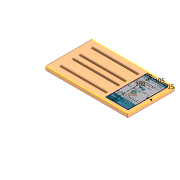
# Autodesk Inventor part: dubpen-platform
Saved by Autodesk Inventor 2020 (Build 240168000, 168)
## iProperties
Created: 2021-06-21
Part Number: dubpen-platform
Material: Generic
Document SubType Name: Modeling
Designer: Aidan Lee
Density: 1 g/cm^3
Appearance: Cherry - Natural Low Gloss
Author: Aidan Lee
Autodesk Inventor part; units mm, degrees
ref_plane "YZ Plane" through (0, 0, 0) normal (1, 0, 0) x (0, 1, 0)
ref_plane "XZ Plane" through (0, 0, 0) normal (0, 1, 0) x (-1, 0, 0)
ref_plane "XY Plane" through (0, 0, 0) normal (0, 0, 1) x (1, 0, 0)
sketch "Sketch1" plane through (0, 0, 0) normal (0, 1, 0) x (-1, 0, 0)
  line L0 (0, 0) -> (-390, 0)
  line L1 (-390, 0) -> (-390, -219)
  line L2 (-390, -219) -> (0, -219)
  line L3 (0, -219) -> (0, 0)
  line L4 (-35, -38.7) -> (-255, -38.7)
  line L5 (-255, -38.7) -> (-255, -30.7)
  line L6 (-255, -30.7) -> (-35, -30.7)
  line L7 (-35, -30.7) -> (-35, -38.7)
  line L8 (-35, -97) -> (-255, -97)
  line L9 (-255, -97) -> (-255, -89)
  line L10 (-255, -89) -> (-35, -89)
  line L11 (-35, -89) -> (-35, -97)
  line L12 (68.8158, -109.5) -> (84.9045, -109.5) construction
  line L13 (-35, -180.3) -> (-255, -180.3)
  line L14 (-255, -180.3) -> (-255, -188.3)
  line L15 (-255, -188.3) -> (-35, -188.3)
  line L16 (-35, -188.3) -> (-35, -180.3)
  line L17 (-35, -122) -> (-255, -122)
  line L18 (-255, -122) -> (-255, -130)
  line L19 (-255, -130) -> (-35, -130)
  line L20 (-35, -130) -> (-35, -122)
  point P0 (0, -109.5)
  point P1 (76.8601, -109.5)
  dimension "d0" = 219
  dimension "d1" = 50.3
  dimension "d2" = 8
  dimension "d3" = 8
  dimension "d4" = 35
  dimension "d6" = 220
  dimension "d7" = 25
  dimension "d8" = 30.7
  dimension "d9" = 30.7
  dimension "d12" = 390
  constraints: 42 end point, 8 symmetric about line, 6 parallel, 4 horizontal, 4 point on line, 3 perpendicular, 2 midpoint, 2 vertical alignment, 1 horizontal alignment
  measures "d0" distance of L2.end L0.start
  measures "d1" distance between parallel lines of L4 L10
  measures "d2" distance of L10.end L8.start
  measures "d3" distance of L6.end L4.start
  measures "d4" distance between parallel lines of L3 L7
  measures "d6" distance of L5.end L6.end
  measures "d7" distance between parallel lines of L8 L17
  measures "d8" distance between parallel lines of L2 L15
  measures "d9" distance between parallel lines of L0 L6
  measures "d12" distance of L0.start L0.end
extrude "Extrusion1" add sketch "Sketch1" along normal blind 18
sketch "Sketch3" plane through (0, 0, 0) normal (0, -1, 0) x (1, 0, 0)
  line L0 (390, -219) -> (0, -219) projected
  line L1 (0, 0) -> (390, 0)
  line L2 (390, 0) -> (390, -219)
  line L3 (390, -219) -> (0, -219)
  line L4 (0, -219) -> (0, 0)
  point P0 (0, -219)
  constraints: 8 end point, 2 parallel, 1 horizontal, 1 perpendicular
extrude "Extrusion2" add sketch "Sketch3" against normal blind 8
sketch "Sketch4" plane through (0, 18, 0) normal (0, 1, 0) x (1, 0, 0)
  line L0 (375, 15) -> (270, 15)
  line L1 (270, 15) -> (270, 204)
  line L2 (270, 204) -> (375, 204)
  line L3 (375, 204) -> (375, 15)
  line L4 (390, 0) -> (390, 219) projected
  line L5 (390, 219) -> (0, 219) projected
  line L6 (0, 0) -> (390, 0) projected
  line L7 (255, 130) -> (255, 122) projected
  line L8 (270, 204) -> (374.9963, 204) construction
  line L9 (374.9963, 204) -> (374.9963, 14.9979) construction
  line L10 (374.9963, 14.9979) -> (270, 14.9979) construction
  line L11 (270, 14.9979) -> (270, 204) construction
  point P0 (375, 109.5)
  point P1 (390, 109.5)
  dimension "d24" = 105
  dimension "d25" = 189
  dimension "d27" = 15
  constraints: 8 end point, 2 midpoint, 2 parallel, 1 horizontal, 1 horizontal alignment, 1 perpendicular, 2 other
  measures "d24" distance of L1.end L2.end
  measures "d25" distance of L0.end L1.end
  measures "d27" distance between parallel lines of L4 L3
body "Solid1"
